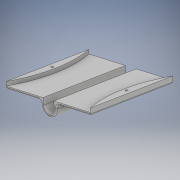
# Autodesk Inventor part: FinalBack
Saved by Autodesk Inventor 2018.3 (Build 223285000, 285)
## iProperties
Created: 2021-06-18
Part Number: FinalBack
Material: Generic
Document SubType Name: Modeling
Designer: Eugene
Density: 1 g/cm^3
Appearance: Default
Author: Eugene
Autodesk Inventor part; units mm, degrees
ref_plane "YZ Plane" through (0, 0, 0) normal (1, 0, 0) x (0, 1, 0)
ref_plane "XZ Plane" through (0, 0, 0) normal (0, 1, 0) x (-1, 0, 0)
ref_plane "XY Plane" through (0, 0, 0) normal (0, 0, 1) x (1, 0, 0)
sketch "Sketch1" plane through (0, 0, 0) normal (0, 1, 0) x (-1, 0, 0)
  line L0 (0, 0) -> (124.865, 0)
  line L1 (124.865, 0) -> (124.865, -120)
  line L2 (124.865, -120) -> (0, -120)
  line L3 (0, -120) -> (0, 0)
  dimension "d0" = 124.865
  dimension "d1" = 120
  constraints: 8 end point, 2 parallel, 1 horizontal, 1 perpendicular
  measures "d0" distance of L1.end L2.end
  measures "d1" distance of L0.end L1.end
extrude "Extrusion1" add sketch "Sketch1" along normal blind 3.5
sketch "Sketch2" plane through (0, 0, 0) normal (0, -1, 0) x (1, 0, 0)
  circle A0 centre (-117.615, -60) radius 1.75
  circle A1 centre (-7.25, -60) radius 1.75
  line L0 (-124.865, 0) -> (-124.865, -120) projected
  line L1 (0, 0) -> (-124.865, 0) projected
  line L2 (0, -120) -> (0, 0) projected
  dimension "d4" = 3.5
  dimension "d5" = 3.5
  dimension "d6" = 7.25
  dimension "d7" = 60
  dimension "d8" = 7.25
  dimension "d9" = 60
  constraints: 2 centre point
  measures "d4" diameter of A0
  measures "d5" diameter of A1
  measures "d6" distance from line of L0 A0.centre
  measures "d7" distance from line of L1 A0.centre
  measures "d8" distance from line of L2 A1.centre
  measures "d9" distance from line of L1 A1.centre
hole "Hole1" at (-7.25, 0, -60) at (-117.615, 0, -60) direction (0, 1, 0) diameter 3.5 end through all countersink diameter 5.5 countersink angle 90
sketch "Sketch3" plane through (0, 0, -120) normal (0, 0, -1) x (-1, 0, 0)
  line L0 (73.933, -5) -> (73.933, 0)
  line L1 (70.433, 0) -> (70.433, -5)
  line L2 (50.933, 0) -> (50.933, -5)
  line L3 (54.433, -5) -> (54.433, 0)
  arc A0 (54.433, -5) -> (70.433, -5) centre (62.433, -5) ccw
  arc A1 (50.933, -5) -> (73.933, -5) centre (62.433, -5) ccw
  line L4 (73.933, 0) -> (73.933, 3.5)
  line L5 (0, 3.5) -> (124.865, 3.5) projected
  line L6 (50.933, 0) -> (50.933, 3.5)
  line L7 (73.933, 3.5) -> (50.933, 3.5)
  line L8 (70.433, 0) -> (54.433, 0)
  line L9 (124.865, 0) -> (0, 0) projected
  dimension "d22" = 3.5
  dimension "d24" = 3.5
  constraints: 16 end point, 4 point on circle, 4 tangent, 2 centre point, 2 collinear, 2 vertical, 1 perpendicular, 1 point on line
  measures "d22" distance between parallel lines of L0 L1
  measures "d24" distance of L2.end L3.start
extrude "Extrusion2" add sketch "Sketch3" against normal blind 120
sketch "Sketch4" plane through (0, 3.5, -120) normal (0, 0, -1) x (-1, 0, 0)
  line L0 (124.865, -3.5) -> (124.865, 0) projected
  line L1 (70.433, -3.5) -> (70.433, -8.5)
  line L2 (54.433, -3.5) -> (54.433, -8.5)
  arc A0 (54.433, -8.5) -> (70.433, -8.5) centre (62.433, -8.5) ccw
  line L3 (70.433, -3.5) -> (70.433, 0)
  line L4 (70.433, 0) -> (54.433, 0)
  line L5 (54.433, 0) -> (54.433, -3.5)
  point P0 (0, -3.5)
  constraints: 10 end point, 2 perpendicular, 2 point on circle, 2 tangent, 1 centre point, 1 vertical
extrude "Extrusion3" cut sketch "Sketch4" against normal blind 120
sketch "Sketch5" plane through (0, 3.5, 0) normal (0, 1, 0) x (1, 0, 0)
  line L0 (0, 120) -> (0, 0) projected
  arc A0 (0, 120) -> (0, 0) centre (138.5716, 60) ccw
  line L1 (-70.433, 120) -> (-124.865, 120) projected
  arc A1 (-124.865, 0) -> (-124.865, 120) centre (-262.4456, 60) ccw
  constraints: 4 point on circle, 2 centre point
extrude "Extrusion4" add sketch "Sketch5" along normal blind 5
sketch "Sketch6" plane through (0, 3.5, 0) normal (0, 1, 0) x (1, 0, 0)
  line L0 (-124.865, 120) -> (-124.865, 0) projected
  arc A0 (-124.865, 0) -> (-124.865, 120) centre (-263.4366, 60) ccw
  point P0 (0, 0)
  constraints: 2 point on circle, 1 centre point
extrude "Extrusion5" add sketch "Sketch6" along normal blind 5
hole "Hole3" at (-117.615, 3.5, -60) direction (0, 1, 0) diameter 3.5 end through all
hole "Hole4" at (-7.2464, 3.5, -59.9915) direction (0, 1, 0) diameter 3.5 end through all
fillet "Fillet2" radius 5 2 edges at (-50.933, 0, -60) (-73.933, 0, -60)
chamfer "Chamfer1" distance 2 angle 45 12 edges at (-124.865, 0, -60) (0, 0, -60) (-62.433, -16.5, -120) (-49.4686, -1.4644, -120) (-22.9665, 0, -120) (-75.3974, -1.4644, -120) (-101.8989, 0, -120) (-62.433, -16.5, 0) (-49.4686, -1.4644, 0) (-22.9665, 0, 0) (-75.3974, -1.4644, 0) (-101.8989, 0, 0)
body "Solid1"
